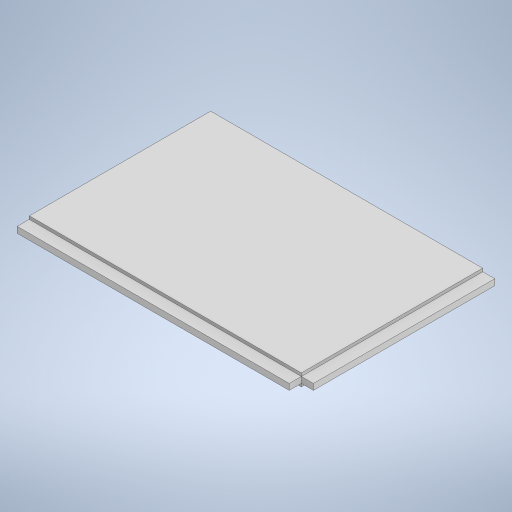
# Autodesk Inventor part: TSU_Baseplate_Male_Cut
Saved by Autodesk Inventor 2024 (Build 280153000, 153)
## iProperties
Created: 2024-12-30
Part Number: TSU_Baseplate_Male_Cut
Material: Generic
Document SubType Name: Modeling
Designer: mtidd
Density: 1 g/cm^3
Appearance: Default
Author: mtidd
Autodesk Inventor part; units mm, degrees
ref_plane "YZ Plane" through (0, 0, 0) normal (1, 0, 0) x (0, 1, 0)
ref_plane "XZ Plane" through (0, 0, 0) normal (0, 1, 0) x (-1, 0, 0)
ref_plane "XY Plane" through (0, 0, 0) normal (0, 0, 1) x (1, 0, 0)
sketch "Sketch1" plane through (0, 0, 0) normal (0, 1, 0) x (-1, 0, 0)
  line L0 (-112.5, 75) -> (112.5, 75)
  line L1 (112.5, 75) -> (112.5, -75)
  line L2 (112.5, -75) -> (-112.5, -75)
  line L3 (-112.5, -75) -> (-112.5, 75)
  line L4 (-112.5, 75) -> (112.5, -75) construction
  line L5 (112.5, 75) -> (-112.5, -75) construction
  point P0 (0, 0)
  dimension "d0" = 225
  dimension "d1" = 150
  constraints: 12 end point, 2 midpoint, 2 parallel, 1 horizontal, 1 perpendicular
  measures "d0" distance of L1.end L2.end
  measures "d1" distance of L0.end L1.end
extrude "Extrusion1" add sketch "Sketch1" along normal blind 10
sketch "Sketch2" plane through (112.5, 0, 75) normal (1, 0, 0) x (0, 0, -1)
  line L0 (0, 2.5) -> (150, 2.5)
  line L1 (150, 2.5) -> (150, 7.5)
  line L2 (150, 7.5) -> (0, 7.5)
  line L3 (0, 7.5) -> (0, 2.5)
  point P0 (75, 0)
  point P1 (0, 5)
  dimension "d4" = 150
  dimension "d5" = 5
  constraints: 8 end point, 2 parallel, 1 horizontal, 1 perpendicular
  measures "d4" distance of L2.end L1.end
  measures "d5" distance of L1.end L0.end
extrude "Extrusion2" add sketch "Sketch2" along normal blind 10
sketch "Sketch3" plane through (-112.5, 0, 75) normal (0, 0, 1) x (1, 0, 0)
  line L0 (0, 2.5) -> (225, 2.5)
  line L1 (225, 2.5) -> (225, 7.5)
  line L2 (225, 7.5) -> (0, 7.5)
  line L3 (0, 7.5) -> (0, 2.5)
  point P0 (112.5, 0)
  dimension "d8" = 225
  dimension "d9" = 5
  constraints: 8 end point, 2 parallel, 1 horizontal, 1 perpendicular
  measures "d8" distance of L2.end L1.end
  measures "d9" distance of L1.end L0.end
extrude "Extrusion3" add sketch "Sketch3" along normal blind 10
body "Solid1"
